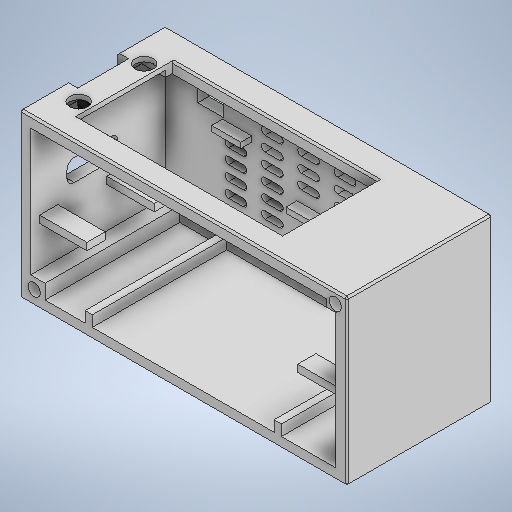
# Autodesk Inventor part: carcaça esboço
Saved by Autodesk Inventor 2025 (Build 290162000, 162)
## iProperties
Created: 2026-04-06
Part Number: carcaça esboço
Material: Genérico
Document SubType Name: Modeling
Designer: pedro
Density: 1 g/cm^3
Appearance: Padrão
Author: pedro
Autodesk Inventor part; units mm, degrees
ref_plane "YZ Plane" through (0, 0, 0) normal (1, 0, 0) x (0, 1, 0)
ref_plane "XZ Plane" through (0, 0, 0) normal (0, 1, 0) x (-1, 0, 0)
ref_plane "XY Plane" through (0, 0, 0) normal (0, 0, 1) x (1, 0, 0)
sketch "Esboço4" plane through (0, 0, 0) normal (0, 0, 1) x (1, 0, 0)
  line L0 (-45, -22.5) -> (45, -22.5)
  line L1 (45, -22.5) -> (45, 22.5)
  line L2 (45, 22.5) -> (-45, 22.5)
  line L3 (-45, 22.5) -> (-45, -22.5)
  line L4 (-45, -22.5) -> (45, 22.5) construction
  line L5 (45, -22.5) -> (-45, 22.5) construction
  line L6 (-45, -22.5) -> (-40, -22.5)
  line L7 (-45, -17.5) -> (-45, -22.5)
  point P0 (0, 0)
  point P1 (40.5, 22.5)
  dimension "d21" = 90
  dimension "d22" = 45
  constraints: 16 end point, 2 horizontal, 2 midpoint, 2 parallel, 1 horizontal alignment, 1 perpendicular
  measures "d21" distance of L1.end L2.end
  measures "d22" distance of L2.end L0.start
extrude "Extrusão3" add sketch "Esboço4" along normal blind 40
shell "Casca4" thickness 3 removed faces 1 at (15, -7.5, 40)
sketch "Esboço6" plane through (-45, 22.5, 0) normal (0, 1, 0) x (1, 0, 0)
  line L0 (9.5, -7.6) -> (65.9, -7.6)
  line L1 (65.9, -7.6) -> (65.9, -33.6)
  line L2 (65.9, -33.6) -> (9.5, -33.6)
  line L3 (9.5, -33.6) -> (9.5, -7.6)
  line L4 (9.5, -7.6) -> (65.9, -33.6) construction
  line L5 (65.9, -7.6) -> (9.5, -33.6) construction
  line L6 (90, 0) -> (0, 0) projected
  line L7 (0, 0) -> (0, -40) projected
  circle A0 centre (6.35, -12.1) radius 2.5
  circle A1 centre (6.35, -30.1) radius 2.5
  line L8 (9.5, -20.6) -> (0, -20.6)
  point P0 (45, 0)
  point P1 (37.7, -20.6)
  dimension "d46" = 56.4
  dimension "d47" = 26
  dimension "d48" = 20.6
  dimension "d49" = 9.5
  dimension "d55" = 5
  dimension "d56" = 5
  dimension "d58" = 18
  dimension "d239" = 3.15
  dimension "d250" = 4.5
  constraints: 14 end point, 3 midpoint, 2 centre point, 2 parallel, 2 perpendicular, 1 horizontal, 1 point on line, 1 vertical alignment
  measures "d46" distance of L0.start L0.end
  measures "d47" distance of L2.end L0.start
  measures "d48" distance from line of L8.start L6
  measures "d49" distance between parallel lines of L7 L3
  measures "d55" diameter of A0
  measures "d56" diameter of A1
  measures "d58" distance of A1.centre A0.centre
  measures "d239" distance from line of L3 A0.centre
  measures "d250" distance from line of L0 A0.centre
extrude "Extrusão5" cut sketch "Esboço6" against normal up to surface (3 mm away)
sketch "Esboço7" plane through (-45, -22.5, 0) normal (-1, 0, 0) x (0, 0, 1)
  line L0 (13.025, 45) -> (27.025, 45)
  line L1 (27.025, 45) -> (27.025, 39)
  line L2 (27.025, 39) -> (13.025, 39)
  line L3 (13.025, 39) -> (13.025, 45)
  line L4 (13.025, 45) -> (27.025, 39) construction
  line L5 (27.025, 45) -> (13.025, 39) construction
  line L6 (0, 45) -> (40, 45) projected
  line L7 (40, 45) -> (40, 0) projected
  line L8 (0, 45) -> (0, 0) projected
  line L9 (33.6, 45) -> (7.6, 45) projected
  line L10 (7.6, 42) -> (33.6, 42) projected
  line L11 (7.6, 45) -> (7.6, 42) projected
  line L12 (33.6, 45) -> (7.6, 45) projected
  line L13 (33.6, 45) -> (33.6, 42) projected
  point P0 (0, 22.5)
  point P1 (20.025, 42)
  point P2 (20.6, 45)
  point P3 (13.025, 42)
  dimension "d50" = 0
  dimension "d51" = 6
  dimension "d60" = 14
  dimension "d220" = 20.025
  constraints: 12 end point, 4 midpoint, 2 parallel, 1 horizontal, 1 perpendicular
  measures "d50" distance between parallel lines of L6 L0
  measures "d51" distance between parallel lines of L2 L0
  measures "d60" distance of L0.start L0.end
  measures "d220" distance from line of L8 point (20.025, 42)
extrude "Extrusão6" cut sketch "Esboço7" against normal blind 3 contours L0 L1 L10 L3 | L10 L1 L2 L3
sketch "Esboço11" plane through (-42, 19.5, 3) normal (0, 0, 1) x (1, 0, 0)
  line L0 (0, -39) -> (84, -39) projected
  line L1 (0, -39) -> (4, -39)
  line L2 (4, -39) -> (4, -35)
  line L3 (4, -35) -> (0, -35)
  line L4 (0, -35) -> (0, -39)
  line L5 (0, 0) -> (84, 0) projected
  line L6 (84, 0) -> (80, 0)
  line L7 (81.5, -2) -> (85.5, -2)
  line L8 (85.5, -2) -> (85.5, 2)
  line L9 (85.5, 2) -> (81.5, 2)
  line L10 (81.5, 2) -> (81.5, -2)
  line L11 (87, 3) -> (-3, 3) projected
  line L12 (87, -42) -> (87, 3) projected
  point P0 (42, -19.5)
  point P1 (4, -37)
  point P2 (2, -35)
  point P3 (83.5, 2)
  point P4 (81.5, 0)
  dimension "d89" = 4
  dimension "d90" = 4
  dimension "d221" = 4
  dimension "d222" = 4
  dimension "d223" = 1
  dimension "d224" = 1.5
  constraints: 18 end point, 4 midpoint, 4 parallel, 3 horizontal, 2 perpendicular
  measures "d89" distance of L3.end L2.end
  measures "d90" distance of L2.end L1.end
  measures "d221" distance of L9.end L8.end
  measures "d222" distance of L8.end L7.end
  measures "d223" distance from line of L11 point (83.5, 2)
  measures "d224" distance between parallel lines of L12 L8
extrude "Extrusão10" add sketch "Esboço11" along normal up to surface (37 mm away)
chamfer "Chanfro3" distance 0.5 angle 45 16 edges at (-45, 22.5, 6.5125) (-45, 22.5, 33.5125) (45, 22.5, 20) (45, -22.5, 20) (-45, -22.5, 20) (0, 22.5, 0) (0, -22.5, 0) (0, 22.5, 40) (0, -22.5, 40) (-45, 0, 40) (-45, 0, 0) (45, 0, 40) (45, 0, 0) (-7.3, 22.5, 7.6) (-7.3, 22.5, 33.6) (20.9, 22.5, 20.6)
sketch "Esboço16" plane through (-42, 16.5, 27.025) normal (1, 0, 0) x (0, 0, -1)
  line L0 (-12.475, 9) -> (26.525, 9) projected
  line L1 (-10.475, -21) -> (-5.475, -21)
  line L2 (-5.475, -21) -> (-5.475, -19)
  line L3 (-5.475, -19) -> (-10.475, -19)
  line L4 (-10.475, -19) -> (-10.475, -21)
  line L5 (8.025, -21) -> (13.025, -21)
  line L6 (13.025, -21) -> (13.025, -19)
  line L7 (13.025, -19) -> (8.025, -19)
  line L8 (8.025, -19) -> (8.025, -21)
  line L9 (-12.975, -38.5) -> (-12.975, 5.5) projected
  line L10 (27.025, 5.5) -> (27.025, -38.5) projected
  line L11 (26.525, -39) -> (-12.475, -39) projected
  point P0 (27.025, -16.5)
  dimension "d146" = 5
  dimension "d147" = 2
  dimension "d148" = 5
  dimension "d150" = 2.5
  dimension "d151" = 14
  dimension "d172" = 18
  constraints: 16 end point, 4 parallel, 2 horizontal, 2 perpendicular, 2 point on line
  measures "d146" distance of L2.end L3.end
  measures "d147" distance of L3.end L1.start
  measures "d148" distance of L6.end L7.end
  measures "d150" distance between parallel lines of L4 L9
  measures "d151" distance between parallel lines of L6 L10
  measures "d172" distance between parallel lines of L11 L1
fillet "Arredondamento1" radius 2 2 edges at (-43.5, 16.5, 13.025) (-43.5, 16.5, 27.025)
sketch "Esboço17" plane through (-45, -22, 0.5) normal (-1, 0, 0) x (0, 0, 1)
  line L0 (17.5, 28.5) -> (27.5, 28.5)
  line L1 (29.5, 26.5) -> (29.5, 24.5)
  line L2 (27.5, 22.5) -> (17.5, 22.5)
  line L3 (15.5, 24.5) -> (15.5, 26.5)
  line L4 (15.5, 28.5) -> (29.5, 22.5) construction
  line L5 (29.5, 28.5) -> (15.5, 22.5) construction
  line L6 (24.525, 38.5) -> (14.525, 38.5) projected
  arc A0 (17.5, 28.5) -> (15.5, 26.5) centre (17.5, 26.5) ccw
  arc A1 (29.5, 26.5) -> (27.5, 28.5) centre (27.5, 26.5) ccw
  arc A2 (27.5, 22.5) -> (29.5, 24.5) centre (27.5, 24.5) ccw
  arc A3 (15.5, 24.5) -> (17.5, 22.5) centre (17.5, 24.5) ccw
  line L7 (0, -0.5) -> (39, -0.5) projected
  line L8 (39.5, 0) -> (39.5, 44) projected
  point P0 (-0.5, 22)
  point P1 (22.5, 25.5)
  point P2 (15.5, 25.5)
  point P3 (19.525, 41.5)
  point P4 (19.525, 38.5)
  point P5 (12.5, 26.5)
  point P6 (26.5, 26.5)
  point P7 (22.5, 28.5)
  dimension "d160" = 6
  dimension "d161" = 14
  dimension "d163" = 2
  dimension "d218" = 29
  dimension "d219" = 17
  constraints: 12 end point, 8 point on circle, 8 point on line, 8 tangent, 5 midpoint, 4 centre point, 3 equal radius, 2 parallel, 1 horizontal, 1 perpendicular
  measures "d160" distance between parallel lines of L2 L0
  measures "d161" distance of L4.start L5.start
  measures "d163" radius of A0
  measures "d218" distance between parallel lines of L7 L0
  measures "d219" distance from line of L8 point (22.5, 28.5)
extrude "Extrusão14" cut sketch "Esboço17" against normal blind 3
sketch "Esboço18" plane through (0, 0, 40) normal (0, 0, 1) x (1, 0, 0)
  line L0 (-38, -19.5) -> (42, -19.5) projected
  line L1 (-27, -19.5) -> (-25, -19.5)
  line L2 (-25, -19.5) -> (-25, -16.5)
  line L3 (-25, -16.5) -> (-27, -16.5)
  line L4 (-27, -16.5) -> (-27, -19.5)
  line L5 (0, -24.4619) -> (0, -28.9958)
  line L6 (27, -19.5) -> (25, -19.5)
  line L7 (25, -19.5) -> (25, -16.5)
  line L8 (25, -16.5) -> (27, -16.5)
  line L9 (27, -16.5) -> (27, -19.5)
  point P0 (0, 0)
  point P1 (25, -18)
  point P2 (-25, -18)
  point P3 (25, -19.5)
  dimension "d166" = 2
  dimension "d167" = 3
  dimension "d168" = 50
  dimension "d169" = 25
  constraints: 18 end point, 4 symmetric about line, 2 midpoint, 2 parallel, 1 horizontal, 1 perpendicular, 1 point on line, 1 vertical
  measures "d166" distance of L3.end L2.end
  measures "d167" distance of L2.end L1.end
  measures "d168" distance of point (25, -18) point (-25, -18)
  measures "d169" distance from line of point (0, 0) L2
extrude "Extrusão15" add sketch "Esboço18" against normal through all
extrude "Extrusão16" add sketch "Esboço16" along normal blind 13
mirror "Espelhar4" about plane through (0, 0, 0) normal (1, 0, 0) of "Extrusão16"
sketch "Esboço19" plane through (-42, 19.5, 3) normal (0, 0, 1) x (1, 0, 0)
  line L0 (36.2644, -29) -> (44.2644, -29)
  line L1 (44.2644, -29) -> (44.2644, -26)
  line L2 (44.2644, -26) -> (36.2644, -26)
  line L3 (36.2644, -26) -> (36.2644, -29)
  line L4 (-2.5, -41.5) -> (-2.5, 2.5) projected
  line L5 (86.5, -41.5) -> (-2.5, -41.5) projected
  line L6 (86.5, 2.5) -> (86.5, -41.5) projected
  line L7 (-2.5, 2.5) -> (86.5, 2.5) projected
  line L8 (15, -36) -> (15, -39) projected
  line L9 (15, -39) -> (4, -39) projected
  line L10 (4, -35) -> (4, -39) projected
  line L11 (0, -35) -> (4, -35) projected
  line L12 (0, -35) -> (0, 0) projected
  line L13 (0, 0) -> (81.5, 0) projected
  line L14 (84, -2) -> (84, -39) projected
  line L15 (84, -39) -> (69, -39) projected
  line L16 (69, -39) -> (69, -36) projected
  line L17 (69, -36) -> (67, -36) projected
  line L18 (67, -36) -> (67, -39) projected
  line L19 (67, -39) -> (17, -39) projected
  line L20 (17, -39) -> (17, -36) projected
  line L21 (17, -36) -> (15, -36) projected
  line L22 (67, -39) -> (17, -39) projected
  line L23 (-2.5, -42) -> (86.5, -42) projected
  line L24 (81.5, -2) -> (81.5, 0) projected
  line L25 (84, -2) -> (81.5, -2) projected
  point P0 (40.2644, -26)
  point P1 (42, -39)
  dimension "d175" = 8
  dimension "d176" = 3
  dimension "d216" = 13
  constraints: 8 end point, 2 midpoint, 1 horizontal, 1 parallel, 1 perpendicular
  measures "d175" distance of L2.end L1.end
  measures "d176" distance of L1.end L0.end
  measures "d216" distance between parallel lines of L23 L0
extrude "Extrusão17" add sketch "Esboço19" along normal blind 8 and the other way blind 2 contours L3 L2 L1 L0
sketch "Esboço20" plane through (0, 0, 0) normal (0, 0, -1) x (-1, 0, 0)
  line L0 (26, 11.5) -> (33, 11.5)
  line L1 (33, 11.5) -> (33, 18.5)
  line L2 (33, 18.5) -> (26, 18.5)
  line L3 (26, 18.5) -> (26, 11.5)
  line L4 (45, -22) -> (45, 22) projected
  line L5 (44.5, 22.5) -> (-44.5, 22.5) projected
  line L6 (-39.5, 14) -> (-35.5, 14) construction
  line L7 (-39.5, 13) -> (-35.5, 13)
  line L8 (-35.5, 15) -> (-39.5, 15)
  arc A0 (-39.5, 15) -> (-39.5, 13) centre (-39.5, 14) ccw
  arc A1 (-35.5, 13) -> (-35.5, 15) centre (-35.5, 14) ccw
  line L9 (-44.5, -22) -> (-44.5, 22) projected
  line L10 (44.5, -22) -> (-44.5, -22) projected
  line L11 (44.5, 22) -> (44.5, -22) projected
  line L12 (-44.5, 22) -> (44.5, 22) projected
  arc A2 (-25.5, 13) -> (-25.5, 15) centre (-25.5, 14) ccw
  line L13 (-29.5, 14) -> (-25.5, 14) construction
  line L14 (-29.5, 13) -> (-25.5, 13)
  line L15 (-25.5, 15) -> (-29.5, 15)
  arc A3 (-29.5, 15) -> (-29.5, 13) centre (-29.5, 14) ccw
  arc A4 (-15.5, 13) -> (-15.5, 15) centre (-15.5, 14) ccw
  line L16 (-19.5, 14) -> (-15.5, 14) construction
  line L17 (-19.5, 13) -> (-15.5, 13)
  line L18 (-15.5, 15) -> (-19.5, 15)
  arc A5 (-19.5, 15) -> (-19.5, 13) centre (-19.5, 14) ccw
  arc A6 (-5.5, 13) -> (-5.5, 15) centre (-5.5, 14) ccw
  line L19 (-9.5, 14) -> (-5.5, 14) construction
  line L20 (-9.5, 13) -> (-5.5, 13)
  line L21 (-5.5, 15) -> (-9.5, 15)
  arc A7 (-9.5, 15) -> (-9.5, 13) centre (-9.5, 14) ccw
  arc A8 (4.5, 13) -> (4.5, 15) centre (4.5, 14) ccw
  line L22 (0.5, 14) -> (4.5, 14) construction
  line L23 (0.5, 13) -> (4.5, 13)
  line L24 (4.5, 15) -> (0.5, 15)
  arc A9 (0.5, 15) -> (0.5, 13) centre (0.5, 14) ccw
  arc A10 (14.5, 13) -> (14.5, 15) centre (14.5, 14) ccw
  line L25 (10.5, 14) -> (14.5, 14) construction
  line L26 (10.5, 13) -> (14.5, 13)
  line L27 (14.5, 15) -> (10.5, 15)
  arc A11 (10.5, 15) -> (10.5, 13) centre (10.5, 14) ccw
  arc A12 (24.5, 13) -> (24.5, 15) centre (24.5, 14) ccw
  line L28 (20.5, 14) -> (24.5, 14) construction
  line L29 (20.5, 13) -> (24.5, 13)
  line L30 (24.5, 15) -> (20.5, 15)
  arc A13 (20.5, 15) -> (20.5, 13) centre (20.5, 14) ccw
  arc A14 (-35.5, 9) -> (-35.5, 11) centre (-35.5, 10) ccw
  line L31 (-39.5, 10) -> (-35.5, 10) construction
  line L32 (-39.5, 9) -> (-35.5, 9)
  line L33 (-35.5, 11) -> (-39.5, 11)
  arc A15 (-39.5, 11) -> (-39.5, 9) centre (-39.5, 10) ccw
  arc A16 (-25.5, 9) -> (-25.5, 11) centre (-25.5, 10) ccw
  line L34 (-29.5, 10) -> (-25.5, 10) construction
  line L35 (-29.5, 9) -> (-25.5, 9)
  line L36 (-25.5, 11) -> (-29.5, 11)
  arc A17 (-29.5, 11) -> (-29.5, 9) centre (-29.5, 10) ccw
  arc A18 (-15.5, 9) -> (-15.5, 11) centre (-15.5, 10) ccw
  line L37 (-19.5, 10) -> (-15.5, 10) construction
  line L38 (-19.5, 9) -> (-15.5, 9)
  line L39 (-15.5, 11) -> (-19.5, 11)
  arc A19 (-19.5, 11) -> (-19.5, 9) centre (-19.5, 10) ccw
  arc A20 (-5.5, 9) -> (-5.5, 11) centre (-5.5, 10) ccw
  line L40 (-9.5, 10) -> (-5.5, 10) construction
  line L41 (-9.5, 9) -> (-5.5, 9)
  line L42 (-5.5, 11) -> (-9.5, 11)
  arc A21 (-9.5, 11) -> (-9.5, 9) centre (-9.5, 10) ccw
  arc A22 (4.5, 9) -> (4.5, 11) centre (4.5, 10) ccw
  line L43 (0.5, 10) -> (4.5, 10) construction
  line L44 (0.5, 9) -> (4.5, 9)
  line L45 (4.5, 11) -> (0.5, 11)
  arc A23 (0.5, 11) -> (0.5, 9) centre (0.5, 10) ccw
  arc A24 (14.5, 9) -> (14.5, 11) centre (14.5, 10) ccw
  line L46 (10.5, 10) -> (14.5, 10) construction
  line L47 (10.5, 9) -> (14.5, 9)
  line L48 (14.5, 11) -> (10.5, 11)
  arc A25 (10.5, 11) -> (10.5, 9) centre (10.5, 10) ccw
  arc A26 (24.5, 9) -> (24.5, 11) centre (24.5, 10) ccw
  line L49 (20.5, 10) -> (24.5, 10) construction
  line L50 (20.5, 9) -> (24.5, 9)
  line L51 (24.5, 11) -> (20.5, 11)
  arc A27 (20.5, 11) -> (20.5, 9) centre (20.5, 10) ccw
  arc A28 (-35.5, 5) -> (-35.5, 7) centre (-35.5, 6) ccw
  line L52 (-39.5, 6) -> (-35.5, 6) construction
  line L53 (-39.5, 5) -> (-35.5, 5)
  line L54 (-35.5, 7) -> (-39.5, 7)
  arc A29 (-39.5, 7) -> (-39.5, 5) centre (-39.5, 6) ccw
  arc A30 (-25.5, 5) -> (-25.5, 7) centre (-25.5, 6) ccw
  line L55 (-29.5, 6) -> (-25.5, 6) construction
  line L56 (-29.5, 5) -> (-25.5, 5)
  line L57 (-25.5, 7) -> (-29.5, 7)
  arc A31 (-29.5, 7) -> (-29.5, 5) centre (-29.5, 6) ccw
  arc A32 (-15.5, 5) -> (-15.5, 7) centre (-15.5, 6) ccw
  line L58 (-19.5, 6) -> (-15.5, 6) construction
  line L59 (-19.5, 5) -> (-15.5, 5)
  line L60 (-15.5, 7) -> (-19.5, 7)
  arc A33 (-19.5, 7) -> (-19.5, 5) centre (-19.5, 6) ccw
  arc A34 (-5.5, 5) -> (-5.5, 7) centre (-5.5, 6) ccw
  line L61 (-9.5, 6) -> (-5.5, 6) construction
  line L62 (-9.5, 5) -> (-5.5, 5)
  line L63 (-5.5, 7) -> (-9.5, 7)
  arc A35 (-9.5, 7) -> (-9.5, 5) centre (-9.5, 6) ccw
  arc A36 (4.5, 5) -> (4.5, 7) centre (4.5, 6) ccw
  line L64 (0.5, 6) -> (4.5, 6) construction
  line L65 (0.5, 5) -> (4.5, 5)
  line L66 (4.5, 7) -> (0.5, 7)
  arc A37 (0.5, 7) -> (0.5, 5) centre (0.5, 6) ccw
  arc A38 (14.5, 5) -> (14.5, 7) centre (14.5, 6) ccw
  line L67 (10.5, 6) -> (14.5, 6) construction
  line L68 (10.5, 5) -> (14.5, 5)
  line L69 (14.5, 7) -> (10.5, 7)
  arc A39 (10.5, 7) -> (10.5, 5) centre (10.5, 6) ccw
  arc A40 (24.5, 5) -> (24.5, 7) centre (24.5, 6) ccw
  line L70 (20.5, 6) -> (24.5, 6) construction
  line L71 (20.5, 5) -> (24.5, 5)
  line L72 (24.5, 7) -> (20.5, 7)
  arc A41 (20.5, 7) -> (20.5, 5) centre (20.5, 6) ccw
  arc A42 (-35.5, 1) -> (-35.5, 3) centre (-35.5, 2) ccw
  line L73 (-39.5, 2) -> (-35.5, 2) construction
  line L74 (-39.5, 1) -> (-35.5, 1)
  line L75 (-35.5, 3) -> (-39.5, 3)
  arc A43 (-39.5, 3) -> (-39.5, 1) centre (-39.5, 2) ccw
  arc A44 (-25.5, 1) -> (-25.5, 3) centre (-25.5, 2) ccw
  line L76 (-29.5, 2) -> (-25.5, 2) construction
  line L77 (-29.5, 1) -> (-25.5, 1)
  line L78 (-25.5, 3) -> (-29.5, 3)
  arc A45 (-29.5, 3) -> (-29.5, 1) centre (-29.5, 2) ccw
  arc A46 (-15.5, 1) -> (-15.5, 3) centre (-15.5, 2) ccw
  line L79 (-19.5, 2) -> (-15.5, 2) construction
  line L80 (-19.5, 1) -> (-15.5, 1)
  line L81 (-15.5, 3) -> (-19.5, 3)
  arc A47 (-19.5, 3) -> (-19.5, 1) centre (-19.5, 2) ccw
  arc A48 (-5.5, 1) -> (-5.5, 3) centre (-5.5, 2) ccw
  line L82 (-9.5, 2) -> (-5.5, 2) construction
  line L83 (-9.5, 1) -> (-5.5, 1)
  line L84 (-5.5, 3) -> (-9.5, 3)
  arc A49 (-9.5, 3) -> (-9.5, 1) centre (-9.5, 2) ccw
  arc A50 (4.5, 1) -> (4.5, 3) centre (4.5, 2) ccw
  line L85 (0.5, 2) -> (4.5, 2) construction
  line L86 (0.5, 1) -> (4.5, 1)
  line L87 (4.5, 3) -> (0.5, 3)
  arc A51 (0.5, 3) -> (0.5, 1) centre (0.5, 2) ccw
  arc A52 (14.5, 1) -> (14.5, 3) centre (14.5, 2) ccw
  line L88 (10.5, 2) -> (14.5, 2) construction
  line L89 (10.5, 1) -> (14.5, 1)
  line L90 (14.5, 3) -> (10.5, 3)
  arc A53 (10.5, 3) -> (10.5, 1) centre (10.5, 2) ccw
  arc A54 (24.5, 1) -> (24.5, 3) centre (24.5, 2) ccw
  line L91 (20.5, 2) -> (24.5, 2) construction
  line L92 (20.5, 1) -> (24.5, 1)
  line L93 (24.5, 3) -> (20.5, 3)
  arc A55 (20.5, 3) -> (20.5, 1) centre (20.5, 2) ccw
  arc A56 (-35.5, -3) -> (-35.5, -1) centre (-35.5, -2) ccw
  line L94 (-39.5, -2) -> (-35.5, -2) construction
  line L95 (-39.5, -3) -> (-35.5, -3)
  line L96 (-35.5, -1) -> (-39.5, -1)
  arc A57 (-39.5, -1) -> (-39.5, -3) centre (-39.5, -2) ccw
  arc A58 (-25.5, -3) -> (-25.5, -1) centre (-25.5, -2) ccw
  line L97 (-29.5, -2) -> (-25.5, -2) construction
  line L98 (-29.5, -3) -> (-25.5, -3)
  line L99 (-25.5, -1) -> (-29.5, -1)
  arc A59 (-29.5, -1) -> (-29.5, -3) centre (-29.5, -2) ccw
  arc A60 (-15.5, -3) -> (-15.5, -1) centre (-15.5, -2) ccw
  line L100 (-19.5, -2) -> (-15.5, -2) construction
  line L101 (-19.5, -3) -> (-15.5, -3)
  line L102 (-15.5, -1) -> (-19.5, -1)
  arc A61 (-19.5, -1) -> (-19.5, -3) centre (-19.5, -2) ccw
  arc A62 (-5.5, -3) -> (-5.5, -1) centre (-5.5, -2) ccw
  line L103 (-9.5, -2) -> (-5.5, -2) construction
  line L104 (-9.5, -3) -> (-5.5, -3)
  line L105 (-5.5, -1) -> (-9.5, -1)
  arc A63 (-9.5, -1) -> (-9.5, -3) centre (-9.5, -2) ccw
  arc A64 (4.5, -3) -> (4.5, -1) centre (4.5, -2) ccw
  line L106 (0.5, -2) -> (4.5, -2) construction
  line L107 (0.5, -3) -> (4.5, -3)
  line L108 (4.5, -1) -> (0.5, -1)
  arc A65 (0.5, -1) -> (0.5, -3) centre (0.5, -2) ccw
  arc A66 (14.5, -3) -> (14.5, -1) centre (14.5, -2) ccw
  line L109 (10.5, -2) -> (14.5, -2) construction
  line L110 (10.5, -3) -> (14.5, -3)
  line L111 (14.5, -1) -> (10.5, -1)
  arc A67 (10.5, -1) -> (10.5, -3) centre (10.5, -2) ccw
  arc A68 (24.5, -3) -> (24.5, -1) centre (24.5, -2) ccw
  line L112 (20.5, -2) -> (24.5, -2) construction
  line L113 (20.5, -3) -> (24.5, -3)
  line L114 (24.5, -1) -> (20.5, -1)
  arc A69 (20.5, -1) -> (20.5, -3) centre (20.5, -2) ccw
  arc A70 (-35.5, -7) -> (-35.5, -5) centre (-35.5, -6) ccw
  line L115 (-39.5, -6) -> (-35.5, -6) construction
  line L116 (-39.5, -7) -> (-35.5, -7)
  line L117 (-35.5, -5) -> (-39.5, -5)
  arc A71 (-39.5, -5) -> (-39.5, -7) centre (-39.5, -6) ccw
  arc A72 (-25.5, -7) -> (-25.5, -5) centre (-25.5, -6) ccw
  line L118 (-29.5, -6) -> (-25.5, -6) construction
  line L119 (-29.5, -7) -> (-25.5, -7)
  line L120 (-25.5, -5) -> (-29.5, -5)
  arc A73 (-29.5, -5) -> (-29.5, -7) centre (-29.5, -6) ccw
  arc A74 (-15.5, -7) -> (-15.5, -5) centre (-15.5, -6) ccw
  line L121 (-19.5, -6) -> (-15.5, -6) construction
  line L122 (-19.5, -7) -> (-15.5, -7)
  line L123 (-15.5, -5) -> (-19.5, -5)
  arc A75 (-19.5, -5) -> (-19.5, -7) centre (-19.5, -6) ccw
  arc A76 (-5.5, -7) -> (-5.5, -5) centre (-5.5, -6) ccw
  line L124 (-9.5, -6) -> (-5.5, -6) construction
  line L125 (-9.5, -7) -> (-5.5, -7)
  line L126 (-5.5, -5) -> (-9.5, -5)
  arc A77 (-9.5, -5) -> (-9.5, -7) centre (-9.5, -6) ccw
  arc A78 (4.5, -7) -> (4.5, -5) centre (4.5, -6) ccw
  line L127 (0.5, -6) -> (4.5, -6) construction
  line L128 (0.5, -7) -> (4.5, -7)
  line L129 (4.5, -5) -> (0.5, -5)
  arc A79 (0.5, -5) -> (0.5, -7) centre (0.5, -6) ccw
  arc A80 (14.5, -7) -> (14.5, -5) centre (14.5, -6) ccw
  line L130 (10.5, -6) -> (14.5, -6) construction
  line L131 (10.5, -7) -> (14.5, -7)
  line L132 (14.5, -5) -> (10.5, -5)
  arc A81 (10.5, -5) -> (10.5, -7) centre (10.5, -6) ccw
  arc A82 (24.5, -7) -> (24.5, -5) centre (24.5, -6) ccw
  line L133 (20.5, -6) -> (24.5, -6) construction
  line L134 (20.5, -7) -> (24.5, -7)
  line L135 (24.5, -5) -> (20.5, -5)
  arc A83 (20.5, -5) -> (20.5, -7) centre (20.5, -6) ccw
  arc A84 (-35.5, -11) -> (-35.5, -9) centre (-35.5, -10) ccw
  line L136 (-39.5, -10) -> (-35, -10) construction
  line L137 (-39.5, -11) -> (-35.5, -11)
  line L138 (-35.5, -9) -> (-39.5, -9)
  arc A85 (-39.5, -9) -> (-39.5, -11) centre (-39.5, -10) ccw
  arc A86 (-25.5, -11) -> (-25.5, -9) centre (-25.5, -10) ccw
  line L139 (-29.5, -10) -> (-25, -10) construction
  line L140 (-29.5, -11) -> (-25.5, -11)
  line L141 (-25.5, -9) -> (-29.5, -9)
  arc A87 (-29.5, -9) -> (-29.5, -11) centre (-29.5, -10) ccw
  arc A88 (-15.5, -11) -> (-15.5, -9) centre (-15.5, -10) ccw
  line L142 (-19.5, -10) -> (-15.5, -10) construction
  line L143 (-19.5, -11) -> (-15.5, -11)
  line L144 (-15.5, -9) -> (-19.5, -9)
  arc A89 (-19.5, -9) -> (-19.5, -11) centre (-19.5, -10) ccw
  arc A90 (-5.5, -11) -> (-5.5, -9) centre (-5.5, -10) ccw
  line L145 (-9.5, -10) -> (-5.5, -10) construction
  line L146 (-9.5, -11) -> (-5.5, -11)
  line L147 (-5.5, -9) -> (-9.5, -9)
  arc A91 (-9.5, -9) -> (-9.5, -11) centre (-9.5, -10) ccw
  arc A92 (4.5, -11) -> (4.5, -9) centre (4.5, -10) ccw
  line L148 (0.5, -10) -> (4.5, -10) construction
  line L149 (0.5, -11) -> (4.5, -11)
  line L150 (4.5, -9) -> (0.5, -9)
  arc A93 (0.5, -9) -> (0.5, -11) centre (0.5, -10) ccw
  arc A94 (14.5, -11) -> (14.5, -9) centre (14.5, -10) ccw
  line L151 (10.5, -10) -> (14.5, -10) construction
  line L152 (10.5, -11) -> (14.5, -11)
  line L153 (14.5, -9) -> (10.5, -9)
  arc A95 (10.5, -9) -> (10.5, -11) centre (10.5, -10) ccw
  arc A96 (24.5, -11) -> (24.5, -9) centre (24.5, -10) ccw
  line L154 (20.5, -10) -> (24.5, -10) construction
  line L155 (20.5, -11) -> (24.5, -11)
  line L156 (24.5, -9) -> (20.5, -9)
  arc A97 (20.5, -9) -> (20.5, -11) centre (20.5, -10) ccw
  point P0 (0, 0)
  point P1 (-37.5, 14)
  point P2 (-27.5, 14)
  point P3 (-17.5, 14)
  point P4 (-7.5, 14)
  point P5 (2.5, 14)
  point P6 (12.5, 14)
  point P7 (22.5, 14)
  point P8 (-37.5, 10)
  point P9 (-27.5, 10)
  point P10 (-17.5, 10)
  point P11 (-7.5, 10)
  point P12 (2.5, 10)
  point P13 (12.5, 10)
  point P14 (22.5, 10)
  point P15 (-37.5, 6)
  point P16 (-27.5, 6)
  point P17 (-17.5, 6)
  point P18 (-7.5, 6)
  point P19 (2.5, 6)
  point P20 (12.5, 6)
  point P21 (22.5, 6)
  point P22 (-37.5, 2)
  point P23 (-27.5, 2)
  point P24 (-17.5, 2)
  point P25 (-7.5, 2)
  point P26 (2.5, 2)
  point P27 (12.5, 2)
  point P28 (22.5, 2)
  point P29 (-37.5, -2)
  point P30 (-27.5, -2)
  point P31 (-17.5, -2)
  point P32 (-7.5, -2)
  point P33 (2.5, -2)
  point P34 (12.5, -2)
  point P35 (22.5, -2)
  point P36 (-37.5, -6)
  point P37 (-27.5, -6)
  point P38 (-17.5, -6)
  point P39 (-7.5, -6)
  point P40 (2.5, -6)
  point P41 (12.5, -6)
  point P42 (22.5, -6)
  point P43 (-37.5, -10)
  point P44 (-27.5, -10)
  point P45 (-17.5, -10)
  point P46 (-7.5, -10)
  point P47 (2.5, -10)
  point P48 (12.5, -10)
  point P49 (22.5, -10)
  dimension "d198" = 7
  dimension "d199" = 7
  dimension "d200" = 12
  dimension "d201" = 4
  dimension "d202" = 4
  dimension "d203" = 2
  dimension "d206" = 10
  dimension "d209" = 4
  dimension "d214" = 7
  dimension "d215" = 7
  constraints: 398 end point, 196 point on circle, 98 centre point, 4 tangent, 3 horizontal, 3 parallel, 2 point on line, 1 midpoint, 1 perpendicular, 1 vertical, 576 other
  measures "d198" distance of L2.end L1.end
  measures "d199" distance of L1.end L0.end
  measures "d200" distance between parallel lines of L4 L1
  measures "d201" distance between parallel lines of L5 L2
  measures "d202" distance of L6.start L6.end
  measures "d203" diameter of A1
  measures "d206" distance of L6.end L13.end
  measures "d209" distance of L6.end L31.end
  measures "d214" distance from line of L9 point (-37.5, 14)
  measures "d215" distance between parallel lines of L12 L8
extrude "Extrusão20" cut sketch "Esboço20" against normal up to surface (3 mm away) contours L3 L2 L1 L0 | A0 L8 A1 L7 | L14 A3 L15 A2 | L17 A5 L18 A4 | L20 A7 L21 A6 | L23 A9 L24 A8 | L26 A11 L27 A10 | L32 A15 L33 A14 | L41 A21 L42 A20 | L44 A23 L45 A22 | L47 A25 L48 A24 | L53 A29 L54 A28 | L56 A31 L57 A30 | L59 A33 L60 A32 | L62 A35 L63 A34 | L65 A37 L66 A36 | L68 A39 L69 A38 | L71 A41 L72 A40 | L74 A43 L75 A42 | L77 A45 L78 A44 | L80 A47 L81 A46 | L83 A49 L84 A48 | L89 A53 L90 A52 | L92 A55 L93 A54 | L95 A57 L96 A56 | L98 A59 L99 A58 | L101 A61 L102 A60 | L104 A63 L105 A62 | L110 A67 L111 A66 | L113 A69 L114 A68 | L116 A71 L117 A70 | L119 A73 L120 A72 | L122 A75 L123 A74 | L125 A77 L126 A76 | L128 A79 L129 A78 | L131 A81 L132 A80 | L134 A83 L135 A82 | L137 A85 L138 A84 | L143 A89 L144 A88 | L146 A91 L147 A90 | L149 A93 L150 A92 | L152 A95 L153 A94
sketch "Esboço21" plane through (0, 0, 40) normal (0, 0, 1) x (1, 0, 0)
  circle A0 centre (-41, -18.5) radius 1.7
  circle A1 centre (41.8, 19.5) radius 1.7
  line L0 (-38, -15.5) -> (-38, -19.5) projected
  line L1 (-42, -15.5) -> (-38, -15.5) projected
  line L2 (45, -22) -> (45, 22) projected
  line L3 (44.5, 22.5) -> (-44.5, 22.5) projected
  point P0 (0, 0)
  point P1 (-38, -17.5)
  dimension "d228" = 3.4
  dimension "d229" = 3.4
  dimension "d230" = 3
  dimension "d231" = 3
  dimension "d232" = 3.2
  dimension "d233" = 3
  constraints: 2 centre point, 1 midpoint
  measures "d228" diameter of A0
  measures "d229" diameter of A1
  measures "d230" horizontal distance of point (-38, -17.5) A0.centre
  measures "d231" distance from line of L1 A0.centre
  measures "d232" distance from line of L2 A1.centre
  measures "d233" distance from line of L3 A1.centre
extrude "Extrusão21" cut sketch "Esboço21" against normal blind 20
sketch "Esboço22" plane through (-44.5, -22.5, 0.5) normal (0, -1, 0) x (1, 0, 0)
  line L0 (83.2542, 25.2937) -> (62.6542, 25.2937)
  line L1 (62.6542, 25.2937) -> (62.6542, 9.6937)
  line L2 (62.6542, 9.6937) -> (83.2542, 9.6937)
  line L3 (83.2542, 9.6937) -> (83.2542, 25.2937)
  point P0 (44.5, -0.5)
  dimension "d248" = 20.6
  dimension "d249" = 15.6
  constraints: 8 end point, 2 parallel, 1 horizontal, 1 perpendicular
  measures "d248" distance of L2.end L1.end
  measures "d249" distance of L0.end L1.end
extrude "Extrusão22" cut sketch "Esboço22" against normal blind 1
sketch "Esboço23" plane through (-42, 19.5, 3) normal (0, 0, 1) x (1, 0, 0)
  line L0 (36.2644, -19.2) -> (44.2644, -19.2)
  line L1 (44.2644, -19.2) -> (44.2644, -17.7)
  line L2 (44.2644, -17.7) -> (36.2644, -17.7)
  line L3 (36.2644, -17.7) -> (36.2644, -19.2)
  line L4 (44.2644, -26) -> (36.2644, -26) projected
  line L5 (86.5, 3) -> (-2.5, 3) projected
  line L6 (15.8, -10) -> (23.8, -10)
  line L7 (23.8, -10) -> (23.8, -8.5)
  line L8 (23.8, -8.5) -> (15.8, -8.5)
  line L9 (15.8, -8.5) -> (15.8, -10)
  line L10 (61.6, -10) -> (69.6, -10)
  line L11 (69.6, -10) -> (69.6, -8.5)
  line L12 (69.6, -8.5) -> (61.6, -8.5)
  line L13 (61.6, -8.5) -> (61.6, -10)
  line L14 (-3, 2.5) -> (-3, -41.5) projected
  point P0 (42, -19.5)
  point P1 (40.2644, -17.7)
  point P2 (40.2644, -26)
  point P3 (11.7602, -11.4003)
  point P4 (19.8, -8.5)
  point P5 (65.6, -8.5)
  point P6 (61.6, -9.25)
  point P7 (23.8, -9.25)
  dimension "d241" = 8
  dimension "d242" = 1.5
  dimension "d243" = 20.7
  dimension "d257" = 8
  dimension "d258" = 1.5
  dimension "d259" = 8
  dimension "d260" = 1.5
  dimension "d261" = 11.5
  dimension "d262" = 18.8
  dimension "d263" = 45.8
  constraints: 24 end point, 6 midpoint, 6 parallel, 3 horizontal, 3 perpendicular, 1 horizontal alignment, 1 vertical alignment
  measures "d241" distance of L2.end L1.end
  measures "d242" distance of L1.end L0.end
  measures "d243" distance between parallel lines of L2 L5
  measures "d257" distance of L8.end L7.end
  measures "d258" distance of L7.end L6.end
  measures "d259" distance of L12.end L11.end
  measures "d260" distance of L11.end L10.end
  measures "d261" distance between parallel lines of L5 L8
  measures "d262" distance between parallel lines of L14 L9
  measures "d263" distance between parallel lines of L9 L13
extrude "Extrusão23" add sketch "Esboço23" along normal blind 3 and the other way blind 1.5
sketch "Esboço24" plane through (-42, 19.5, 3) normal (0, -1, 0) x (1, 0, 0)
  line L0 (-0.0477, 30.4225) -> (5.5422, 30.4225)
  line L1 (5.4523, 6.4227) -> (-0.0477, 6.4227)
  line L2 (-0.0477, 6.4227) -> (-0.0477, 30.4225)
  circle A0 centre (3.35, 27.1) radius 2.5 projected
  circle A1 centre (3.35, 9.1) radius 2.5 projected
  line L3 (6.5, 31.1) -> (6.5, 4.1) projected
  line L4 (5.4523, 6.4227) -> (6.5, 6.4227)
  line L5 (6.5, 30.4225) -> (5.5422, 30.4225)
  point P0 (42, -3)
  point P1 (5.85, 27.1)
  point P2 (5.85, 9.1)
  point P3 (2.7472, 30.4225)
  point P4 (5.8239, 27.4606)
  point P5 (5.7871, 8.5427)
  point P6 (1.1774, 10.025)
  point P7 (5.8226, 10.025)
  dimension "d251" = 5.5
  dimension "d252" = 24
  constraints: 10 end point, 2 point on line, 1 collinear, 1 horizontal, 1 midpoint, 1 parallel, 1 perpendicular, 1 point on circle, 1 vertical, 2 other
  measures "d251" distance of L1.start L1.end
  measures "d252" distance of L0.end L1.start
extrude "Extrusão24" cut sketch "Esboço24" against normal blind 1.7 contours L0 L5 L3 L4 L1 L2 | A1
